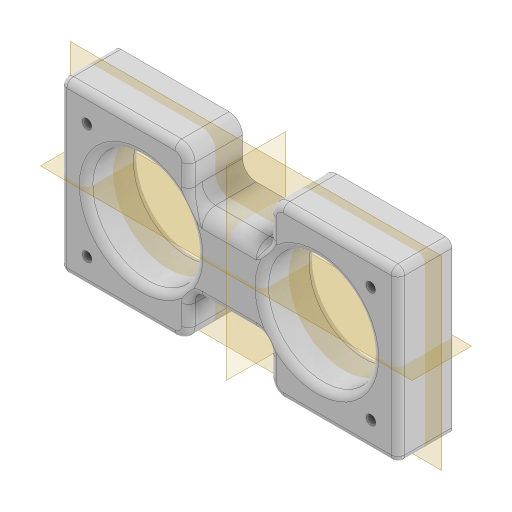
# Autodesk Inventor part: Крепление_ультразвука
Saved by Autodesk Inventor 2023.2 (Build 272271030, 271C)
## iProperties
Created: 2025-05-24
Part Number: Крепление_ультразвука
Material: Типовые
Document SubType Name: Modeling
Designer: Олег Коноваленко
Density: 1 g/cm^3
Appearance: По умолчанию
Author: Олег Коноваленко
Autodesk Inventor part; units mm, degrees
sketch "Эскиз1" plane through (0, 0, 0) normal (0, 0, 1) x (1, 0, 0)
  line L0 (-25, 12.5) -> (25, 12.5)
  line L1 (25, 12.5) -> (25, -12.5)
  line L2 (25, -12.5) -> (-25, -12.5)
  line L3 (-25, -12.5) -> (-25, 12.5)
  line L4 (-25, -12.5) -> (25, 12.5) construction
  line L5 (25, -12.5) -> (-25, 12.5) construction
  point P0 (0, 0)
  point P1 (0, 0)
  dimension "d2" = 50
  dimension "d3" = 25
  constraints: 12 end point, 2 parallel, 1 coincident, 1 horizontal, 1 midpoint, 1 perpendicular
  measures "d2" distance of L0.start L0.end
  measures "d3" distance of L2.end L0.start
extrude "Выдавливание1" add sketch "Эскиз1" along normal mid plane 8
sketch "Эскиз2" plane through (0, 0, 4) normal (0, 0, 1) x (1, 0, 0)
  line L0 (-25, -12.5) -> (25, -12.5) projected
  line L1 (-6, -12.5) -> (6, -12.5)
  line L2 (6, -12.5) -> (6, -5.5)
  line L3 (6, -5.5) -> (-6, -5.5)
  line L4 (-6, -5.5) -> (-6, -12.5)
  line L5 (0, 17.5) -> (0, -17.5) projected
  point P0 (0, 0)
  point P1 (6, -12.5)
  point P2 (0, -5.5)
  dimension "d4" = 7
  dimension "d5" = 12
  constraints: 8 end point, 2 parallel, 2 point on line, 1 horizontal, 1 midpoint, 1 perpendicular
  measures "d4" distance of L3.end L1.start
  measures "d5" distance of L2.end L3.end
extrude "Выдавливание2" cut sketch "Эскиз2" against normal up to next
fillet "Сопряжение1" radius 2 4 edges at (-6, -5.5, 0) (6, -5.5, 0) (6, -12.5, 0) (-6, -12.5, 0)
sketch "Эскиз3" plane through (0, 0, 4) normal (0, 0, 1) x (1, 0, 0)
  circle A0 centre (13, 0.0001) radius 8 projected
  circle A1 centre (-13, 0.0001) radius 8 projected
  circle A2 centre (-13, 0.0001) radius 8.15
  circle A3 centre (13, 0.0001) radius 8.15
  point P0 (0, 0)
  dimension "d22" = 16.3
  dimension "d23" = 16.3
  constraints: 2 centre point, 2 coincident
  measures "d22" diameter of A2
  measures "d23" diameter of A3
extrude "Выдавливание3" cut sketch "Эскиз3" against normal up to next contours A0 | A1 | A2 | A3
sketch "Эскиз4" plane through (0, 0, 4) normal (0, 0, 1) x (1, 0, 0)
  circle A0 centre (21.0274, -8.5002) radius 0.9099 projected
  circle A1 centre (20.984, 8.496) radius 0.9099 projected
  circle A2 centre (-21.0095, 8.4358) radius 0.9099 projected
  circle A3 centre (-20.98, -8.5791) radius 0.9099 projected
  circle A4 centre (-21.0095, 8.4358) radius 0.7
  circle A5 centre (-20.98, -8.5791) radius 0.7
  circle A6 centre (20.984, 8.496) radius 0.7
  circle A7 centre (21.0274, -8.5002) radius 0.7
  dimension "d28" = 1.4
  constraints: 4 centre point, 4 coincident, 3 equal radius
  measures "d28" diameter of A4
extrude "Выдавливание4" cut sketch "Эскиз4" against normal up to next contours A4 | A5 | A6 | A7
sketch "Эскиз5" plane through (0, 0, 4) normal (0, 0, 1) x (1, 0, 0)
  line L0 (-6, 12.5) -> (6, 12.5)
  line L1 (6, 12.5) -> (6, 5.5)
  line L2 (6, 5.5) -> (-6, 5.5)
  line L3 (-6, 5.5) -> (-6, 12.5)
  line L4 (0, 5.5) -> (0, 12.5) construction
  line L5 (0, 17.5) -> (0, -17.5) projected
  line L6 (25, 12.5) -> (-25, 12.5) projected
  point P0 (0, 12.5)
  dimension "d16" = 12
  dimension "d17" = 7
  constraints: 10 end point, 4 midpoint, 2 parallel, 1 horizontal, 1 perpendicular, 1 point on line, 1 vertical
  measures "d16" distance between parallel lines of L1 L3
  measures "d17" distance between parallel lines of L2 L0
extrude "Выдавливание5" cut sketch "Эскиз5" against normal up to next
fillet "Сопряжение2" radius 2 5 edges at (-6, 5.5, 0) (6, 5.5, 0) (-6, 12.5, 0) (6, 12.5, 0) (0, 5.5, 4)
fillet "Сопряжение3" radius 1 4 edges at (-25, 12.5, 0) (-25, -12.5, 0) (25, 12.5, 0) (25, -12.5, 0)
fillet "Сопряжение4" radius 1 4 edges at (-21.15, 0.0001, -4) (-21.15, 0.0001, 4) (4.85, 0.0001, -4) (4.85, 0.0001, 4)
fillet "Сопряжение5" radius 1 23 edges at (5.4142, -6.0858, 4) (6, -9, 4) (6.5858, -11.9142, 4) (16, -12.5, 4) (24.7071, -12.2071, 4) (25, 0, 4) (24.7071, 12.2071, 4) (16, 12.5, 4) (6.5858, 11.9142, 4) (6, 8.7321, 4) (5.3445, 5.0321, 4) (-5.4142, -6.0858, 4) (-6, -9, 4) (-6.5858, -11.9142, 4) (-16, -12.5, 4) (-24.7071, -12.2071, 4) (-25, 0, 4) (-24.7071, 12.2071, 4) (-16, 12.5, 4) (-6.5858, 11.9142, 4) (-6, 8.7321, 4) (-5.3445, 5.0321, 4) (0, -5.5, 4)
sketch "Эскиз6" plane through (0, 0, -4) normal (0, 0, -1) x (-1, 0, 0)
  circle A0 centre (-20.984, 8.496) radius 0.7 projected
  circle A1 centre (-20.984, 8.496) radius 1.2
  circle A2 centre (-21.0274, -8.5002) radius 0.7 projected
  circle A3 centre (-21.0274, -8.5002) radius 1.2
  circle A4 centre (21.0095, 8.4358) radius 0.7 projected
  circle A5 centre (21.0095, 8.4358) radius 1.2
  circle A6 centre (20.98, -8.5791) radius 0.7 projected
  circle A7 centre (20.98, -8.5791) radius 1.2
  point P0 (0, 0)
  dimension "d29" = 2.4
  constraints: 4 centre point, 4 coincident, 3 equal radius
  measures "d29" diameter of A1
extrude "Выдавливание6" cut sketch "Эскиз6" against normal up to surface (4 mm away) contours A0 | A1 | A2 | A3 | A4 | A5 | A6 | A7
